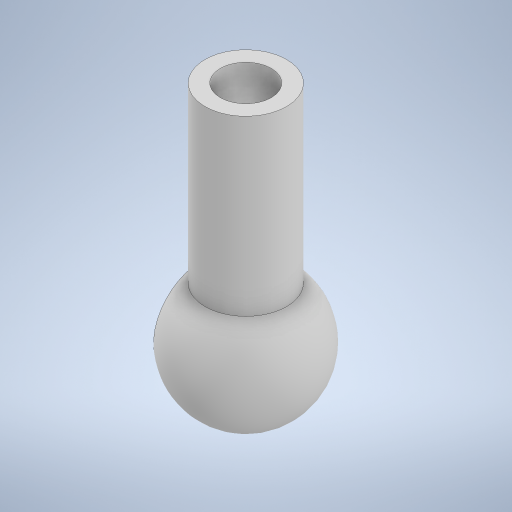
# Autodesk Inventor part: Ball Joint_bot
Saved by Autodesk Inventor 2024 (Build 280153000, 153)
## iProperties
Created: 2024-03-12
Part Number: Ball Joint_bot
Material: 일반
Document SubType Name: Modeling
Designer: unney
Density: 1 g/cm^3
Appearance: 기본값
Author: unney
Autodesk Inventor part; units mm, degrees
ref_plane "YZ Plane" through (0, 0, 0) normal (1, 0, 0) x (0, 1, 0)
ref_plane "XZ Plane" through (0, 0, 0) normal (0, 1, 0) x (-1, 0, 0)
ref_plane "XY Plane" through (0, 0, 0) normal (0, 0, 1) x (1, 0, 0)
sketch "스케치1" plane through (0, 0, 0) normal (0, 0, 1) x (1, 0, 0)
  circle A0 centre (0, 0) radius 6.4
  line L0 (0, 6.4) -> (0, -6.4)
  dimension "d0" = 12.8
  constraints: 2 end point, 2 point on circle, 1 centre point, 1 coincident, 1 vertical
  measures "d0" diameter of A0
sketch "스케치1 outline for SR sphere" plane through (0, 0, 0) normal (0, 0, 1) x (1, 0, 0)
  line L0 (0, 6.4) -> (0, -6.4)
  arc A0 (0, -6.4) -> (0, 6.4) centre (0, 0) ccw
revolve "SR sphere" add sketch "스케치1 outline for SR sphere" angle 360 about axis through (0, 6.4, 0) along (0, -1, 0)
sketch "e" plane through (0, 0, 0) normal (1, 0, 0) x (0, 1, 0)
  circle A0 centre (0, 0) radius 4.647459
  constraints: 1 centre point, 1 coincident
sketch "e outline for e hole" plane through (0, 0, 0) normal (1, 0, 0) x (0, 1, 0)
  circle A0 centre (0, 0) radius 4.647459
extrude "e hole" cut sketch "e outline for e hole" against normal blind 6.4
sketch "스케치6" plane through (0, 0, 0) normal (0, 0, 1) x (1, 0, 0)
  arc A0 (-4.400128, -4.647459) -> (-4.400128, 4.647459) centre (0, 0) ccw
  line L0 (4.001417, 4.994864) -> (4.001417, 21.987002)
  line L1 (4.001417, 21.987002) -> (2.501417, 21.987002)
  line L2 (2.501417, 21.987002) -> (2.501417, 5.890918)
  line L3 (0.001417, -6.4) -> (0.001417, 19.355985)
  line L4 (10.301781, -0.012998) -> (-6.695287, -0.012998)
  line L5 (4.001417, 4.994864) -> (2.501417, 5.890918)
  point P0 (3.251417, 21.987002)
  dimension "d4" = 1.5
  dimension "d5" = 4
  dimension "d6" = 22
  constraints: 12 end point, 3 point on circle, 2 perpendicular, 2 vertical, 1 horizontal, 1 midpoint
  measures "d4" distance of L0.end L1.end
  measures "d5" distance between parallel lines of L3 L0
  measures "d6" distance from line of point (3.251, 21.987) L4
sketch "스케치6 outline for h, g 고려 회전" plane through (0, 0, 0) normal (0, 0, 1) x (1, 0, 0)
  line L0 (4.001417, 21.987002) -> (2.501417, 21.987002)
  line L1 (4.001417, 4.994864) -> (4.001417, 21.987002)
  arc A0 (2.501417, 5.890918) -> (4.001417, 4.994864) centre (0, 0) cw
  line L2 (2.501417, 21.987002) -> (2.501417, 5.890918)
revolve "h, g 고려 회전" add sketch "스케치6 outline for h, g 고려 회전" angle 360 about axis through (0.001417, -6.4, 0) along (0, 1, 0)
